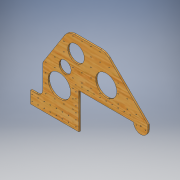
# Autodesk Inventor part: Cote droit Rammasse-Balle
Saved by Autodesk Inventor 2016 (Build 200138000, 138)
## iProperties
Created: 2016-01-24
Part Number: Cote droit Rammasse-Balle
Material: Generic
Document SubType Name: Modeling
Designer: ares-b02
Density: 1 g/cm^3
Appearance: Plywood - New
Author: ares-b02
Autodesk Inventor part; units mm, degrees
ref_plane "YZ Plane" through (0, 0, 0) normal (1, 0, 0) x (0, 1, 0)
ref_plane "XZ Plane" through (0, 0, 0) normal (0, 1, 0) x (-1, 0, 0)
ref_plane "XY Plane" through (0, 0, 0) normal (0, 0, 1) x (1, 0, 0)
sketch "Sketch1" plane through (0, 0, 0) normal (0, 0, 1) x (1, 0, 0)
  line L0 (-644.6123, 24.5323) -> (-426.4123, 367.2389)
  line L1 (-426.4123, 367.2389) -> (-151.4123, 97.5421)
  line L2 (-151.4123, 97.5421) -> (-151.4123, 77.5421)
  line L3 (-644.6123, 24.5323) -> (-644.6123, -73.2577)
  line L4 (-644.6123, -73.2577) -> (-441.4123, -73.2577)
  line L5 (-441.4123, -73.2577) -> (-441.4123, 77.5421)
  line L6 (-441.4123, 77.5421) -> (-211.4123, 77.5421)
  arc A0 (-211.4123, 77.5421) -> (-151.4123, 77.5421) centre (-181.4123, 77.5421) ccw
  circle A1 centre (-181.4123, 77.5421) radius 2.5
  dimension "d0" = 30
  dimension "d1" = 5
  dimension "d2" = 230
  dimension "d3" = 203.2
  dimension "d4" = 150.7998
  dimension "d7" = 97.79
  dimension "d8" = 20
  dimension "d9" = 290.0849
  dimension "d10" = 245
  constraints: 14 end point, 3 perpendicular, 2 centre point, 2 point on circle, 2 vertical, 1 coincident, 1 tangent
  measures "d0" radius of A0
  measures "d1" diameter of A1
  measures "d2" distance of L5.end L6.end
  measures "d3" distance of L3.end L4.end
  measures "d4" distance of L4.end L5.end
  measures "d7" distance of L0.start L3.end
  measures "d8" distance of L1.end L2.end
  measures "d9" distance of L5.end L0.end
  measures "d10" horizontal distance of A0.centre L0.end
extrude "Extrusion1" add sketch "Sketch1" along normal blind 6.35
sketch "Sketch4" plane through (0, 0, 6.35) normal (0, 0, 1) x (1, 0, 0)
  line L0 (-629.5637, 473.3889) -> (-232.1986, 473.3889)
  line L1 (-232.1986, 473.3889) -> (-232.1986, 272.5421)
  line L2 (-232.1986, 272.5421) -> (-629.5637, 272.5421)
  line L3 (-629.5637, 272.5421) -> (-629.5637, 473.3889)
  circle A0 centre (-181.4123, 77.5421) radius 2.5 projected
  point P0 (0, 0)
  dimension "d14" = 397.3651
  dimension "d15" = 200.8468
  dimension "d16" = 195
  dimension "d17" = 50.7863
  constraints: 8 end point, 2 parallel, 1 horizontal, 1 perpendicular
  measures "d14" distance of L0.start L0.end
  measures "d15" distance of L0.end L1.end
  measures "d16" vertical distance of A0.centre L1.end
  measures "d17" horizontal distance of A0.centre L1.end
extrude "Extrusion3" cut sketch "Sketch4" against normal through all contours L0 L1 L2 L3
fillet "Fillet1" radius 50 2 edges at (-329.8534, 272.5421, 3.175) (-486.7054, 272.5421, 3.175)
hole "Hole9" at (-523.9623, 53.7423, 6.35) direction (0, 0, -1) diameter 95.25 end through all
hole "Hole10" at (-326.6141, 153.7421, 6.35) direction (0, 0, -1) diameter 88.9 end through all
hole "Hole11" at (-453.5552, 206.3751, 6.35) direction (0, 0, -1) diameter 69.85 end through all
hole "Hole12" at (-499.6331, 134.0048, 6.35) direction (0, 0, -1) diameter 50.8 end through all
hole "Hole13" at (-428.7123, 96.5921, 6.35) direction (0, 0, -1) diameter 3.175 end through all
pattern_linear "Rectangular Pattern1" count 9 spacing 25.4 along (1, 0, 0) of "Hole13"
hole "Hole14" at (-454.1123, -60.5577, 6.35) direction (0, 0, -1) diameter 3.175 end through all
pattern_linear "Rectangular Pattern2" count 7 spacing 25.4 along (0, 1, 0) of "Hole14"
hole "Hole15" at (-638.2623, -60.5577, 6.35) direction (0, 0, -1) diameter 3.175 end through all
pattern_linear "Rectangular Pattern4" count 7 spacing 25.4 along (1, 0, 0) count 2 spacing 25.4 along (0, 1, 0) of "Hole15"
sketch "Sketch5" plane through (0, 0, 6.35) normal (0, 0, 1) x (1, 0, 0)
  line L0 (-644.6123, -73.2577) -> (-441.4123, -73.2577) projected
  line L1 (-644.6123, 104.5423) -> (-593.8123, 104.5423)
  line L2 (-593.8123, 104.5423) -> (-593.8123, -22.4577)
  line L3 (-593.8123, -22.4577) -> (-644.6123, -22.4577)
  line L4 (-644.6123, -22.4577) -> (-644.6123, 104.5423)
  line L5 (-644.6123, 24.5323) -> (-644.6123, -73.2577) projected
  point P0 (0, 0)
  dimension "d180" = 50.8
  dimension "d181" = 0
  dimension "d182" = 50.8
  dimension "d183" = 127
  constraints: 8 end point, 2 parallel, 1 horizontal, 1 perpendicular
  measures "d180" distance of L2.end L3.end
  measures "d181" distance between parallel lines of L5 L4
  measures "d182" distance between parallel lines of L3 L0
  measures "d183" distance of L3.end L1.start
extrude "Extrusion4" cut sketch "Sketch5" against normal blind 25.4
fillet "Fillet2" radius 25.4 1 edges at (-593.8123, -22.4577, 3.175)
fillet "Fillet3" radius 25.4 1 edges at (-593.8123, 104.3192, 3.175)
hole "Hole17" at (-581.1123, -3.4077, 6.35) direction (0, 0, -1) diameter 3.175 end through all
pattern_linear "Rectangular Pattern5" count 12 spacing 38.1 along (1, 0, 0) count 8 spacing 38.1 along (0, 1, 0) of "Hole17"
body "Solid1"
